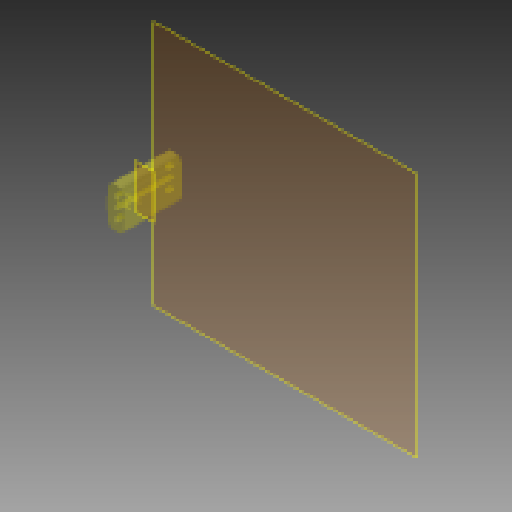
# Autodesk Inventor part: крепление ручки
Saved by Autodesk Inventor 2023 (Build 270158000, 158)
## iProperties
Created: 2025-04-14
Part Number: крепление ручки
Material: Типовые
Document SubType Name: Modeling
Designer: Ivan
Density: 1 g/cm^3
Appearance: Прозрачный — желтый
Author: Ivan
Autodesk Inventor part; units mm, degrees
ref_plane "YZ Plane" through (0, 0, 0) normal (1, 0, 0) x (0, 1, 0)
ref_plane "XZ Plane" through (0, 0, 0) normal (0, 1, 0) x (-1, 0, 0)
ref_plane "XY Plane" through (0, 0, 0) normal (0, 0, 1) x (1, 0, 0)
ref_plane "РабПлоскость1" through (0, 0, 0) normal (0, 0, 1) x (1, 0, 0)
sketch "Эскиз1" plane through (0, 0, 0) normal (0, 0, 1) x (1, 0, 0)
  arc A0 (-36.9892, 97.1998) -> (-36.9892, -97.1998) centre (0, 0) ccw projected
  line L0 (-145.6, 0) -> (145.6, 0) construction
  line L1 (-102.5171, 17.5) -> (-89.5171, 17.5)
  line L2 (-89.5171, 17.5) -> (-89.5171, -17.5)
  line L3 (-89.5171, -17.5) -> (-102.5171, -17.5)
  line L4 (-102.5171, -17.5) -> (-102.5171, 17.5) construction
  line L5 (-104, 0) -> (-89.5171, 0) construction
  circle A1 centre (-96.7585, 0) radius 1.8
  point P0 (0, 0)
  point P1 (-102.5171, 0)
  dimension "d0" = 35
  dimension "d1" = 13
  dimension "d2" = 3.6
  constraints: 12 end point, 3 midpoint, 2 horizontal, 2 parallel, 2 point on circle, 2 point on line, 1 centre point, 1 perpendicular, 2 other
  measures "d0" distance of L3.end L1.start
  measures "d1" distance of L2.end L3.end
  measures "d2" diameter of A1
ref_plane "РабПлоскость2" through (-75.9237, -75.9237, 50) normal (0, 0, 1) x (0.7071068, -0.7071068, 0)
extrude "Выдавливание1" add sketch "Эскиз1" along normal up to surface (50 mm away)
fillet "Сопряжение1" radius 5 4 edges at (-102.5171, 17.5, 25) (-89.5171, 17.5, 25) (-89.5171, -17.5, 25) (-102.5171, -17.5, 25)
sketch "Эскиз2" plane through (-89.5171, -12.5, 0) normal (1, 0, 0) x (0, 0, -1)
  line L0 (-50, 14.3) -> (-50, 10.7) projected
  line L1 (0, 10.7) -> (0, 14.3) projected
  circle A0 centre (-44, 12.5) radius 1
  line L2 (-50, 10.7) -> (0, 10.7) projected
  circle A1 centre (-35, 12.5) radius 1
  line L3 (-50, 12.5) -> (0, 12.5) construction
  line L4 (-50, 25) -> (-50, 0) projected
  point P0 (0, 12.5)
  dimension "d6" = 2
  dimension "d9" = 6
  dimension "d10" = 15
  constraints: 3 midpoint, 2 centre point, 2 end point, 2 point on line, 1 equal radius
  measures "d6" diameter of A0
  measures "d9" distance from line of A0.centre L4
  measures "d10" distance from line of A1.centre L4
extrude "Выдавливание2" cut sketch "Эскиз2" against normal through all
chamfer "Фаска1" distance 1.3 angle 45 2 edges at (-104, 0.0084, 45) (-104, 0.0084, 36)
sketch "Эскиз3" plane through (-98.2077, -17.5, 50) normal (0, 0, 1) x (1, 0, 0)
  line L0 (1.4492, 35) -> (1.4492, 0) construction
  circle A0 centre (1.4492, 17.5) radius 1.8 projected
  line L1 (0, 35) -> (3.6906, 35) construction
  line L2 (3.6906, 0) -> (0, 0) construction
  circle A1 centre (1.4492, 26.25) radius 1.9
  circle A2 centre (1.4492, 8.75) radius 1.9
  point P0 (98.2077, 17.5)
  point P1 (1.4492, 17.5)
  dimension "d16" = 17.5
  dimension "d17" = 8.75
  dimension "d18" = 8.75
  dimension "d19" = 3.8
  constraints: 4 point on line, 3 coincident, 2 centre point, 2 end point, 2 midpoint, 1 equal radius, 1 vertical
  measures "d16" distance from line of point (1.449, 17.5) L1
  measures "d17" distance from line of point (1.449, 26.25) L1
  measures "d18" distance from line of point (1.449, 8.75) L2
  measures "d19" diameter of A1
extrude "Выдавливание3" cut sketch "Эскиз3" against normal blind 5.5 contours A1 | A2
ref_plane "РабПлоскость3" through (-98.2077, -17.5, 25) normal (0, 0, 1) x (1, 0, 0)
mirror "Зеркальное отражение1" about plane through (-98.2077, -17.5, 25) normal (0, 0, 1) of "Выдавливание3"
equation "\"d17\" = 0.5 * d16"
equation "\"d18\" = d17"
